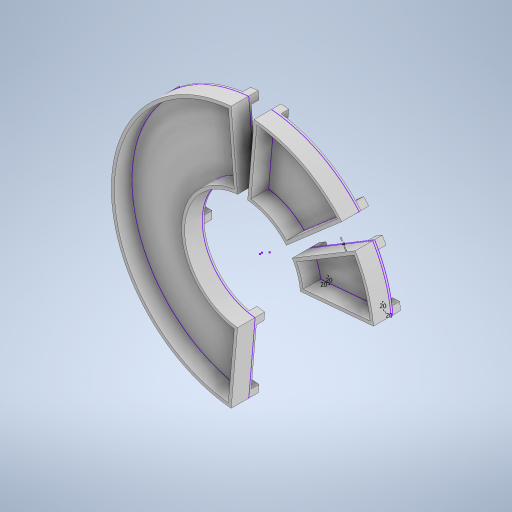
# Autodesk Inventor part: Bandeja Radial
Saved by Autodesk Inventor 2023 (Build 270158000, 158)
## iProperties
Created: 2023-03-08
Part Number: Bandeja Radial
Material: Genérico
Document SubType Name: Modeling
Designer: Inteli
Density: 1 g/cm^3
Appearance: Padrão
Author: Inteli
Autodesk Inventor part; units mm, degrees
ref_plane "YZ Plane" through (0, 0, 0) normal (1, 0, 0) x (0, 1, 0)
ref_plane "XZ Plane" through (0, 0, 0) normal (0, 1, 0) x (-1, 0, 0)
ref_plane "XY Plane" through (0, 0, 0) normal (0, 0, 1) x (1, 0, 0)
sketch "Esboço1" plane through (0, 0, 0) normal (0, 0, 1) x (1, 0, 0)
  line L0 (-13.0734, -149.4292) -> (-29.633, -338.7062)
  line L1 (-13.0734, 149.4292) -> (-29.633, 338.7062)
  line L2 (13.0734, 149.4292) -> (29.633, 338.7062)
  line L3 (149.4292, 13.0734) -> (338.7062, 29.633)
  arc A0 (-29.633, 338.7062) -> (-29.633, -338.7062) centre (0, 0) ccw
  arc A1 (-13.0734, 149.4292) -> (-13.0734, -149.4292) centre (0, 0) ccw
  line L4 (113.2064, 98.4089) -> (256.6013, 223.0601)
  line L5 (128.5751, 77.2557) -> (291.4369, 175.1129)
  arc A2 (338.7062, 29.633) -> (291.4369, 175.1129) centre (0, 0) ccw
  arc A3 (256.6013, 223.0601) -> (29.633, 338.7062) centre (0, 0) ccw
  arc A4 (149.4292, 13.0734) -> (128.5751, 77.2557) centre (0, 0) ccw
  arc A5 (113.2064, 98.4089) -> (13.0734, 149.4292) centre (0, 0) ccw
  line L6 (-36.8969, 329.9434) -> (-21.7225, 156.4996)
  arc A6 (-21.7225, 156.4996) -> (-21.7225, -156.4996) centre (0, 0) ccw
  line L7 (-21.7225, -156.4996) -> (-36.8969, -329.9434)
  arc A7 (-36.8969, 329.9434) -> (-36.8969, -329.9434) centre (0, 0) ccw
  line L8 (36.8969, 329.9434) -> (21.7225, 156.4996)
  arc A8 (113.8427, 109.562) -> (21.7225, 156.4996) centre (0, 0) ccw
  line L9 (113.8427, 109.562) -> (245.2424, 223.786)
  arc A9 (245.2424, 223.786) -> (36.8969, 329.9434) centre (0, 0) ccw
  line L10 (288.6172, 164.0857) -> (139.379, 74.4143)
  arc A10 (156.4996, 21.7225) -> (139.379, 74.4143) centre (0, 0) ccw
  line L11 (156.4996, 21.7225) -> (329.9434, 36.8969)
  arc A11 (329.9434, 36.8969) -> (288.6172, 164.0857) centre (0, 0) ccw
  constraints: 24 end point, 24 point on circle, 12 centre point, 1 coincident, 9 other
extrude "Parede" add sketch "Esboço1" along normal blind 45
extrude "Fundo" add sketch "Esboço1" against normal blind 5 contours L0 A0 L1 A1 | L2 A3 L4 A5 | A4 L5 A2 L3 | L6 A6 L7 A7 | A9 L9 A8 L8 | A11 L11 A10 L10
sketch "Esboço3" plane through (0, 0, -5) normal (0, 0, -1) x (-1, 0, 0)
  arc A0 (-29.633, 338.7062) -> (-338.7062, 29.633) centre (0, 0) ccw projected
  line L0 (247.3834, 233.2412) -> (233.3452, 219.2031)
  line L1 (233.2412, 247.3834) -> (219.2031, 233.3452)
  arc A1 (233.3452, 219.2031) -> (219.2031, 233.3452) centre (0.1105, 0.1105) ccw
  arc A2 (247.3834, 233.2412) -> (233.2412, 247.3834) centre (0, 0) ccw
  line L2 (170, 0) -> (170, -10)
  line L3 (170, -10) -> (149.6663, -10)
  line L4 (170, 0) -> (170, 10)
  line L5 (170, 10) -> (149.6648, 10.0224)
  arc A3 (149.6663, -10) -> (149.6648, 10.0224) centre (0, 0) ccw
  line L6 (320, 0) -> (320, -10)
  line L7 (320, 0) -> (320, 10)
  line L8 (320, 10) -> (339.8529, 10)
  line L9 (320, -10) -> (339.8529, -10)
  arc A4 (339.8529, -10) -> (339.8529, 10) centre (0, 0) ccw
  line L10 (247.3834, -233.2412) -> (233.3452, -219.2031)
  line L11 (233.2412, -247.3834) -> (219.2031, -233.3452)
  arc A5 (219.2031, -233.3452) -> (233.3452, -219.2031) centre (0.1105, -0.1105) ccw
  arc A6 (233.2412, -247.3834) -> (247.3834, -233.2412) centre (0, 0) ccw
  arc A7 (29.633, -338.7062) -> (29.633, 338.7062) centre (0, 0) ccw projected
  line L12 (29.633, 338.7062) -> (27.8898, 318.7823)
  line L13 (27.8898, 318.7823) -> (47.8137, 317.0392)
  line L14 (47.8137, 317.0392) -> (49.5055, 336.3766)
  arc A8 (49.5055, 336.3766) -> (29.633, 338.7062) centre (0, 0) ccw
  line L15 (13.0734, 149.4292) -> (14.8165, 169.3531)
  line L16 (14.8165, 169.3531) -> (34.7404, 167.61)
  line L17 (34.7404, 167.61) -> (32.8805, 146.3519)
  arc A9 (13.0734, -149.4292) -> (13.0734, 149.4292) centre (0, 0) ccw projected
  arc A10 (32.8805, 146.3519) -> (13.0734, 149.4292) centre (0, 0) ccw
  line L18 (29.633, -338.7062) -> (27.8898, -318.7823)
  line L19 (27.8898, -318.7823) -> (47.8137, -317.0392)
  line L20 (47.8137, -317.0392) -> (49.5055, -336.3766)
  arc A11 (29.633, -338.7062) -> (49.5055, -336.3766) centre (0, 0) ccw
  line L21 (13.0734, -149.4292) -> (14.8165, -169.3531)
  line L22 (14.8165, -169.3531) -> (34.7404, -167.61)
  line L23 (34.7404, -167.61) -> (32.8805, -146.3519)
  arc A12 (13.0734, -149.4292) -> (32.8805, -146.3519) centre (0, 0) ccw
  dimension "d58" = 20
  dimension "d59" = 20
  dimension "d60" = 20
  constraints: 48 end point, 24 point on circle, 10 centre point, 6 perpendicular, 2 vertical, 1 concentric, 1 parallel, 2 other
  measures "d58" distance of L12.start L12.end
  measures "d59" distance of L12.end L13.end
  measures "d60" distance of L15.start L15.end
extrude "Pé da Bandeja G" add sketch "Esboço3" along normal blind 20
sketch "Esboço5" plane through (0, 0, -5) normal (0, 0, -1) x (-1, 0, 0)
  line L0 (-13.0734, 149.4292) -> (-14.8165, 169.3531)
  line L1 (-14.8165, 169.3531) -> (-34.7404, 167.61)
  line L2 (-34.7404, 167.61) -> (-32.8838, 146.3888)
  arc A0 (-13.0734, 149.4292) -> (-113.2064, 98.4089) centre (0, 0) ccw projected
  arc A1 (-13.0734, 149.4292) -> (-32.8838, 146.3888) centre (1.0004, -8.3311) ccw
  line L3 (-256.6013, 223.0601) -> (-113.2064, 98.4089) projected
  line L4 (-113.2064, 98.4089) -> (-128.3006, 111.53)
  line L5 (-128.3006, 111.53) -> (-115.1794, 126.6242)
  line L6 (-115.1794, 126.6242) -> (-99.0745, 112.6244)
  arc A2 (-99.0745, 112.6244) -> (-113.2064, 98.4089) centre (0, 0) ccw
  line L7 (-29.633, 338.7062) -> (-27.8898, 318.7823)
  line L8 (-27.8898, 318.7823) -> (-47.8137, 317.0392)
  line L9 (-47.8137, 317.0392) -> (-49.5055, 336.3766)
  line L10 (-256.6013, 223.0601) -> (-241.5071, 209.9389)
  line L11 (-241.5071, 209.9389) -> (-228.3859, 225.0331)
  line L12 (-228.3859, 225.0331) -> (-243.0357, 237.768)
  arc A3 (-243.0357, 237.768) -> (-256.6013, 223.0601) centre (0, 0) ccw
  line L13 (-13.0734, 149.4292) -> (-29.633, 338.7062) projected
  arc A4 (-29.633, 338.7062) -> (-256.6013, 223.0601) centre (0, 0) ccw projected
  arc A5 (-29.633, 338.7062) -> (-49.5055, 336.3766) centre (0, 0) ccw
  dimension "d73" = 20
  dimension "d74" = 20
  dimension "d75" = 20
  constraints: 24 end point, 9 point on circle, 8 perpendicular, 4 centre point, 2 point on line, 1 concentric
  measures "d73" distance of L0.end L1.end
  measures "d74" distance of L3.end L4.end
  measures "d75" distance of L4.end L5.end
extrude "Pé da Bandeja M" add sketch "Esboço5" along normal blind 20 contours A0 A1 L2 L1 L0 | L8 L9 A4 L7 | A0 L3 L5 L6 | L12 L11 L3 A3
sketch "Esboço6" plane through (0, 0, -5) normal (0, 0, -1) x (-1, 0, 0)
  line L0 (-149.4292, 13.0734) -> (-338.7062, 29.633) projected
  line L1 (-149.4292, 13.0734) -> (-169.3531, 14.8165)
  line L2 (-169.3531, 14.8165) -> (-167.61, 34.7404)
  line L3 (-167.61, 34.7404) -> (-146.2196, 32.869)
  arc A0 (-128.5751, 77.2557) -> (-149.4292, 13.0734) centre (0, 0) ccw projected
  line L4 (-338.7062, 29.633) -> (-318.7823, 27.8898)
  line L5 (-318.7823, 27.8898) -> (-317.0392, 47.8137)
  line L6 (-317.0392, 47.8137) -> (-336.3766, 49.5055)
  arc A1 (-291.4369, 175.1129) -> (-338.7062, 29.633) centre (0, 0) ccw projected
  line L7 (-128.5751, 77.2557) -> (-291.4369, 175.1129)
  line L8 (-128.5751, 77.2557) -> (-145.7184, 87.5565)
  line L9 (-145.7184, 87.5565) -> (-156.0192, 70.4131)
  line L10 (-156.0192, 70.4131) -> (-137.614, 59.3542)
  line L11 (-274.2935, 164.8122) -> (-284.5943, 147.6688)
  line L12 (-284.5943, 147.6688) -> (-301.233, 157.6664)
  arc A2 (-128.5751, 77.2557) -> (-137.614, 59.3542) centre (-19.7094, 11.0542) ccw
  line L13 (-169.3531, 14.8165) -> (-318.7823, 27.8898)
  line L14 (-291.4369, 175.1129) -> (-128.5751, 77.2557) projected
  line L15 (-128.5751, 77.2557) -> (-291.4369, 175.1129)
  arc A3 (-291.4369, 175.1129) -> (-338.7062, 29.633) centre (0, 0) ccw
  arc A4 (-128.5751, 77.2557) -> (-149.4292, 13.0734) centre (0, 0) ccw
  arc A5 (-141.1866, 61.5008) -> (-150.3716, 33.2322) centre (0, 0) ccw
  line L16 (-169.0045, 18.8013) -> (-318.4337, 31.8746)
  arc A6 (-297.7983, 155.6026) -> (-332.3848, 49.1563) centre (0, 0) ccw
  line L17 (-276.3537, 161.3835) -> (-147.7786, 84.1278)
  line L18 (-147.7786, 84.1278) -> (-145.7184, 87.5565)
  line L19 (-141.1866, 61.5008) -> (-137.7278, 59.4226)
  line L20 (-146.3519, 32.8805) -> (-150.3716, 33.2322)
  line L21 (-169.0045, 18.8013) -> (-169.3531, 14.8165)
  line L22 (-318.7823, 27.8898) -> (-318.4337, 31.8746)
  line L23 (-332.3848, 49.1563) -> (-336.3766, 49.5055)
  line L24 (-297.7983, 155.6026) -> (-301.233, 157.6664)
  point P0 (-301.233, 157.6664)
  point P1 (-291.4369, 175.1129)
  point P2 (-146.3519, 32.8805)
  point P3 (-132.964, 69.4304)
  dimension "d85" = 20
  dimension "d86" = 20
  dimension "d88" = 20
  dimension "d89" = 20
  dimension "d93" = 4
  constraints: 46 end point, 16 point on line, 14 point on circle, 5 centre point, 5 collinear, 3 perpendicular
  measures "d85" distance of L1.end L0.start
  measures "d86" distance of L1.end L2.end
  measures "d88" distance of L4.end L0.end
  measures "d89" distance of L4.end L5.end
  measures "d93" distance between parallel lines of L14 L17
extrude "Pé da Bandeja P" add sketch "Esboço6" along normal blind 20 contours L0 L2 L3 A0 | L0 A1 L6 L5 | L10 L9 L7 A2 A0 | A1 L7 L11 L12
